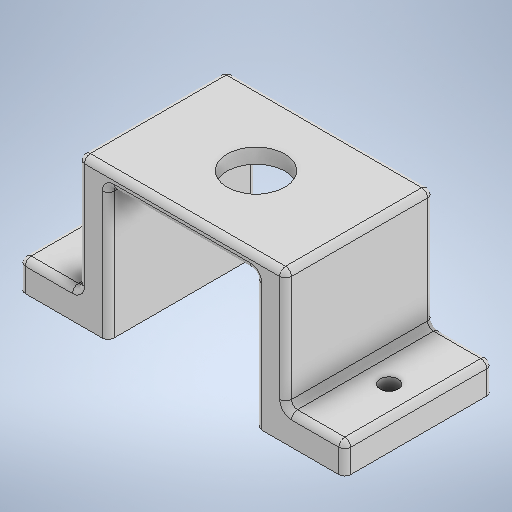
# Autodesk Inventor part: Part2
Saved by Autodesk Inventor 2026.1 (Build 301233000, 233)
## iProperties
Created: 2026-05-22
Part Number: Part2
Material: Generic
Document SubType Name: Modeling
Designer: chris
Density: 1 g/cm^3
Appearance: Default
Author: chris
Autodesk Inventor part; units mm, degrees
ref_plane "YZ Plane" through (0, 0, 0) normal (1, 0, 0) x (0, 1, 0)
ref_plane "XZ Plane" through (0, 0, 0) normal (0, 1, 0) x (-1, 0, 0)
ref_plane "XY Plane" through (0, 0, 0) normal (0, 0, 1) x (1, 0, 0)
sketch "Sketch1" plane through (0, 0, 0) normal (0, 1, 0) x (-1, 0, 0)
  line L0 (55, 25) -> (-55, 25)
  line L1 (-55, 25) -> (-55, -25)
  line L2 (-55, -25) -> (55, -25)
  line L3 (55, -25) -> (55, 25)
  line L4 (55, 25) -> (-55, -25) construction
  line L5 (-55, 25) -> (55, -25) construction
  line L6 (-25, 25) -> (25, 25)
  line L7 (25, 25) -> (25, -25)
  line L8 (25, -25) -> (-25, -25)
  line L9 (-25, -25) -> (-25, 25)
  line L10 (-25, 25) -> (25, -25) construction
  line L11 (25, 25) -> (-25, -25) construction
  point P0 (0, 0)
  dimension "d0" = 110
  dimension "d1" = 50
  dimension "d2" = 50
  dimension "d3" = 50
  constraints: 24 end point, 4 midpoint, 4 parallel, 2 horizontal, 2 perpendicular
  measures "d0" distance of L2.end L1.end
  measures "d1" distance of L1.end L0.end
  measures "d2" distance of L7.end L8.end
  measures "d3" distance of L6.end L7.end
extrude "Extrusion1" add sketch "Sketch1" along normal blind 10 contours L3 L2 L7 L0 | L9 L2 L1 L0
sketch "Sketch2" plane through (0, 10, 0) normal (0, 1, 0) x (1, 0, 0)
  line L0 (-35, -25) -> (-25, -25)
  line L1 (-25, -25) -> (-25, 25)
  line L2 (-25, 25) -> (-35, 25)
  line L3 (-35, 25) -> (-35, -25)
  line L4 (-35, -25) -> (-25, 25) construction
  line L5 (-25, -25) -> (-35, 25) construction
  line L6 (25, -25) -> (35, -25)
  line L7 (35, -25) -> (35, 25)
  line L8 (35, 25) -> (25, 25)
  line L9 (25, 25) -> (25, -25)
  line L10 (25, -25) -> (35, 25) construction
  line L11 (35, -25) -> (25, 25) construction
  line L12 (-25, -25) -> (-25, 25) projected
  line L13 (25, 25) -> (25, -25) projected
  point P0 (0, 0)
  point P1 (-30, 0)
  point P2 (30, 0)
  dimension "d6" = 10
  dimension "d7" = 50
  dimension "d8" = 10
  dimension "d9" = 50
  constraints: 24 end point, 4 midpoint, 4 parallel, 2 collinear, 2 horizontal, 2 perpendicular
  measures "d6" distance of L2.end L1.end
  measures "d7" distance of L1.end L0.end
  measures "d8" distance of L8.end L7.end
  measures "d9" distance of L7.end L6.end
extrude "Extrusion2" add sketch "Sketch2" along normal blind 40
sketch "Sketch3" plane through (0, 50, 0) normal (0, 1, 0) x (1, 0, 0)
  line L0 (-25, -25) -> (25, -25)
  line L1 (25, -25) -> (25, 25)
  line L2 (25, 25) -> (-25, 25)
  line L3 (-25, 25) -> (-25, -25)
  line L4 (-25, -25) -> (25, 25) construction
  line L5 (25, -25) -> (-25, 25) construction
  line L6 (25, 25) -> (25, -25) projected
  line L7 (35, 25) -> (25, 25) projected
  point P0 (0, 0)
  constraints: 12 end point, 2 collinear, 2 midpoint, 2 parallel, 1 horizontal, 1 perpendicular
extrude "Extrusion3" add sketch "Sketch3" against normal blind 5
sketch "Sketch4" plane through (0, 50, 0) normal (0, 1, 0) x (1, 0, 0)
  circle A0 centre (0, 0) radius 9.75
  dimension "d14" = 19.5
  constraints: 1 centre point, 1 coincident
  measures "d14" diameter of A0
extrude "Extrusion4" cut sketch "Sketch4" against normal blind 5
sketch "Sketch5" plane through (0, 10, 0) normal (0, 1, 0) x (1, 0, 0)
  circle A0 centre (-45, 0) radius 3.05
  circle A1 centre (45, 0) radius 3.05
  line L0 (55, -25) -> (55, 25) projected
  line L1 (-55, 25) -> (-55, -25) projected
  point P0 (0, 0)
  dimension "d17" = 6.1
  dimension "d18" = 6.1
  dimension "d22" = 10
  dimension "d23" = 10
  constraints: 2 centre point, 2 horizontal alignment
  measures "d17" diameter of A0
  measures "d18" diameter of A1
  measures "d22" distance from line of L0 A1.centre
  measures "d23" distance from line of L1 A0.centre
extrude "Extrusion5" cut sketch "Sketch5" against normal through all
fillet "Fillet1" radius 2 28 edges at (-55, 10, 0) (-35, 10, 0) (-35, 50, 0) (35, 50, 0) (35, 10, 0) (55, 10, 0) (45, 10, 25) (45, 10, -25) (55, 5, 25) (55, 5, -25) (-45, 10, 25) (-55, 5, 25) (-55, 5, -25) (-45, 10, -25) (35, 30, 25) (35, 30, -25) (0, 50, -25) (0, 50, 25) (-35, 30, 25) (-35, 30, -25) (-25, 22.5, -25) (-25, 22.5, 25) (25, 22.5, -25) (25, 22.5, 25) (0, 45, 25) (0, 45, -25) (-25, 45, 0) (25, 45, 0)
body "Solid1"
